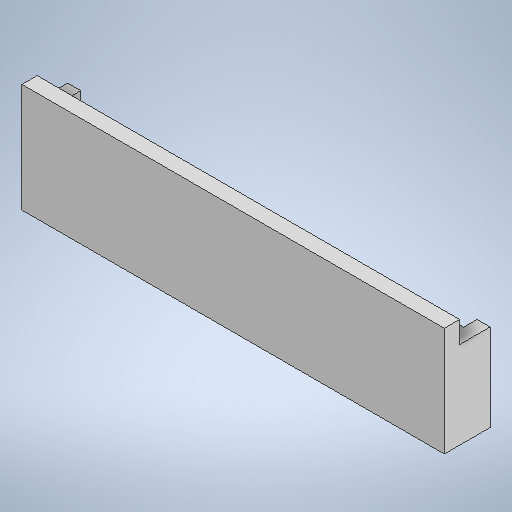
# Autodesk Inventor part: plate holder
Saved by Autodesk Inventor 2025.1 (Build 291241020, 241B)
## iProperties
Created: 2024-12-05
Part Number: plate holder
Material: Generic
Document SubType Name: Modeling
Designer: Hunter Mathis
Density: 1 g/cm^3
Appearance: Default
Author: Hunter Mathis
Autodesk Inventor part; units mm, degrees
ref_plane "YZ Plane" through (0, 0, 0) normal (1, 0, 0) x (0, 1, 0)
ref_plane "XZ Plane" through (0, 0, 0) normal (0, 1, 0) x (-1, 0, 0)
ref_plane "XY Plane" through (0, 0, 0) normal (0, 0, 1) x (1, 0, 0)
sketch "Sketch1" plane through (0, 0, 0) normal (0, 1, 0) x (-1, 0, 0)
  line L0 (61.595, -2.2225) -> (-61.595, -2.2225)
  line L1 (-61.595, -2.2225) -> (-61.595, 2.2225)
  line L2 (-61.595, 2.2225) -> (61.595, 2.2225)
  line L3 (61.595, 2.2225) -> (61.595, -2.2225)
  line L4 (61.595, -2.2225) -> (-61.595, 2.2225) construction
  line L5 (-61.595, -2.2225) -> (61.595, 2.2225) construction
  point P0 (0, 0)
  dimension "d0" = 123.19
  dimension "d1" = 4.445
  constraints: 12 end point, 2 midpoint, 2 parallel, 1 horizontal, 1 perpendicular
  measures "d0" distance of L1.end L2.end
  measures "d1" distance of L0.end L1.end
extrude "Extrusion1" add sketch "Sketch1" along normal blind 31.75
sketch "Sketch2" plane through (61.595, 0, -2.2225) normal (0, 0, -1) x (-1, 0, 0)
  line L0 (123.19, 0) -> (0, 0) projected
  line L1 (0, 0) -> (123.19, 0)
  line L2 (123.19, 0) -> (123.19, 25.4116)
  line L3 (123.19, 25.4116) -> (0, 25.4116)
  line L4 (0, 25.4116) -> (0, 0)
  point P0 (61.595, 0)
  constraints: 8 end point, 3 equal length, 1 perpendicular
extrude "Extrusion2" add sketch "Sketch2" along normal blind 8.89
sketch "Sketch3" plane through (-61.595, 25.4116, -2.2225) normal (0, 1, 0) x (1, 0, 0)
  point P0 (61.595, -2.2225)
sketch "Sketch4" plane through (61.595, 0, -11.1125) normal (0, 0, -1) x (-1, 0, 0)
  line L0 (0, 25.4116) -> (0, 0) projected
  line L1 (3.81, 12.7058) -> (3.81, 25.4116)
  line L2 (0, 25.4116) -> (3.81, 25.4116)
  line L3 (0, 25.4116) -> (0, 12.7058)
  line L4 (0, 12.7058) -> (0, 3.1808)
  line L5 (0, 0) -> (0, 31.75) projected
  line L6 (0, 3.1808) -> (3.81, 3.1808)
  line L7 (3.81, 3.1808) -> (3.81, 12.7058)
  line L8 (0, 25.4116) -> (123.19, 25.4116) projected
  line L9 (123.19, 0) -> (123.19, 25.4116) projected
  line L10 (119.38, 12.7058) -> (119.38, 25.4116)
  line L11 (3.81, 25.4116) -> (119.38, 25.4116)
  line L12 (119.38, 12.7058) -> (119.38, 3.1808)
  line L13 (119.38, 3.1808) -> (123.19, 3.1808)
  line L14 (123.19, 3.1808) -> (123.19, 25.4116)
  line L15 (123.19, 0) -> (123.19, 31.75) projected
  line L16 (3.81, 3.1808) -> (119.38, 3.1808)
  line L17 (3.81, 3.1808) -> (3.81, 15.8808)
  line L18 (119.38, 15.8808) -> (3.81, 15.8808)
  line L19 (119.38, 15.8808) -> (119.38, 3.1808)
  line L20 (3.81, 3.1808) -> (119.38, 3.1808)
  point P0 (61.595, 0)
  dimension "d6" = 3.81
  dimension "d7" = 9.525
  dimension "d13" = 3.81
  dimension "d14" = 12.7
  constraints: 32 end point, 5 collinear, 5 point on line, 4 perpendicular, 1 horizontal, 1 midpoint, 1 parallel, 1 vertical
  measures "d6" distance of L3.end L1.start
  measures "d7" distance of L3.end L4.end
  measures "d13" distance of L12.end L13.end
  measures "d14" distance between parallel lines of L18 L16
extrude "Extrusion3" cut sketch "Sketch4" against normal blind 3.8862 contours L8 L10 L18 L1 | L18 L10 L12 L16 L7 L1
extrude "Extrusion4" add sketch "Sketch4" against normal blind 1.143 contours L18 L10 L12 L16 L7 L1
body "Solid1"
